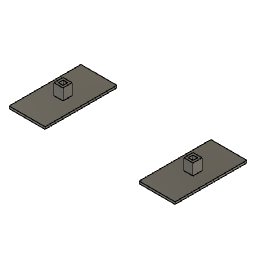
Base of Stand v7 (Autodesk Fusion 360 design; units mm, degrees)
Autodesk Fusion 360 part; units mm, degrees
sketch "Sketch1" plane through (0, 0, 0) normal (0, 0, 1) x (1, 0, 0)
  line L0 (48.9309, 100) -> (358.9309, 100)
  line L1 (358.9309, 100) -> (358.9309, 79.8)
  line L2 (358.9309, 79.8) -> (48.9309, 79.8)
  line L3 (48.9309, 79.8) -> (48.9309, 100)
  line L4 (53.9309, 95) -> (64.1309, 95)
  line L5 (64.1309, 95) -> (64.1309, 84.8)
  line L6 (64.1309, 84.8) -> (53.9309, 84.8)
  line L7 (53.9309, 84.8) -> (53.9309, 95)
  line L8 (69.1309, 100) -> (69.1309, 79.8)
  line L9 (343.7309, 95) -> (353.9309, 95)
  line L10 (353.9309, 95) -> (353.9309, 84.8)
  line L11 (353.9309, 84.8) -> (343.7309, 84.8)
  line L12 (343.7309, 84.8) -> (343.7309, 95)
  line L13 (338.7309, 100) -> (338.7309, 79.8)
  line L14 (338.7309, 92.4) -> (338.7309, 87.4)
  line L15 (69.1309, 87.4) -> (69.1309, 92.4)
  line L16 (18.9309, 170) -> (99.1309, 170)
  line L17 (99.1309, 170) -> (99.1309, 9.8)
  line L18 (99.1309, 9.8) -> (18.9309, 9.8)
  line L19 (18.9309, 9.8) -> (18.9309, 170)
  line L20 (308.7309, 170) -> (388.9309, 170)
  line L21 (388.9309, 170) -> (388.9309, 9.8)
  line L22 (388.9309, 9.8) -> (308.7309, 9.8)
  line L23 (308.7309, 9.8) -> (308.7309, 170)
  dimension "d1" = 310
  dimension "d2" = 20.2
  dimension "d3" = 20.2
  dimension "d4" = 5
  dimension "d5" = 5
  dimension "d6" = 5
  dimension "d7" = 5
  dimension "d8" = 20.2
  dimension "d9" = 20.2
  dimension "d10" = 5
  dimension "d11" = 5
  dimension "d12" = 5
  dimension "d13" = 5
  dimension "d17" = 70
  dimension "d18" = 30
  dimension "d19" = 70
  dimension "d20" = 30
  dimension "d21" = 70
  dimension "d22" = 70
  dimension "d23" = 30
  dimension "d24" = 30
  constraint horizontal L0
  constraint vertical L1
  constraint horizontal L2
  constraint vertical L3
  constraint horizontal L4
  constraint vertical L5
  constraint horizontal L6
  constraint vertical L7
  constraint coincident L0 L8.start
  constraint coincident L2 L8.end
  constraint perpendicular L2 L8
  constraint horizontal L9
  constraint vertical L10
  constraint horizontal L11
  constraint vertical L12
  constraint coincident L0 L13.start
  constraint coincident L2 L13.end
  constraint perpendicular L2 L13
  constraint vertical L14
  constraint vertical L15
  constraint coincident L13 L14.end
  constraint coincident L8 L15.end
  constraint horizontal L16
  constraint vertical L17
  constraint horizontal L18
  constraint vertical L19
  constraint horizontal L20
  constraint vertical L21
  constraint horizontal L22
  constraint vertical L23
  measures "d1" distance of L1 L3
  measures "d2" distance of L0.start L2.end
  measures "d3" distance of L3 L8
  measures "d4" distance of L5 L8
  measures "d5" distance of L0 L4
  measures "d6" distance of L3 L7
  measures "d7" distance of L2 L6
  measures "d8" distance of L0.end L1.end
  measures "d9" distance of L1 L13
  measures "d10" distance of L0 L9
  measures "d11" distance of L1 L10
  measures "d12" distance of L2 L11
  measures "d13" distance of L12 L13
  measures "d17" distance of L0 L16
  measures "d18" distance of L8 L17
  measures "d19" distance of L2 L18
  measures "d20" distance of L3 L19
  measures "d21" distance of L0 L20
  measures "d22" distance of L2 L22
  measures "d23" distance of L1 L21
  measures "d24" distance of L13 L23
extrude "Extrude1" add sketch "Sketch1" along normal blind 2.5 contours L4 L5 L6 L7 | L9 L10 L11 L12 makes body 1 at (57.3309, 88.2, 0) makes body 2 at (347.1309, 91.6, 0)
extrude "Extrude2" add sketch "Sketch1" along normal blind 30 contours L0 L2 L3 L8 L15 | L0 L1 L2 L13 L14 bodies 1 2
extrude "Extrude3" add sketch "Sketch1" along normal blind 5 contours L0 L2 L3 L16 L17 L18 L19 | L0 L2 L8 L15 L17 | L0 L1 L2 L20 L21 L22 L23 | L0 L2 L13 L14 L23 bodies 1 2
